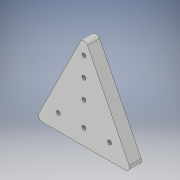
# Autodesk Inventor part: backsupportplate
Saved by Autodesk Inventor 2018 (Build 220112000, 112)
## iProperties
Created: 2018-07-30
Part Number: backsupportplate
Material: Generic
Document SubType Name: Modeling
Designer: Cole Tucker
Density: 1 g/cm^3
Appearance: Default
Author: Cole Tucker
Autodesk Inventor part; units mm, degrees
ref_plane "YZ Plane" through (0, 0, 0) normal (1, 0, 0) x (0, 1, 0)
ref_plane "XZ Plane" through (0, 0, 0) normal (0, 1, 0) x (-1, 0, 0)
ref_plane "XY Plane" through (0, 0, 0) normal (0, 0, 1) x (1, 0, 0)
sketch "Sketch1" plane through (0, 0, 0) normal (0, 0, 1) x (1, 0, 0)
  line L0 (0, 0) -> (0, 76.2)
  line L1 (0, 0) -> (32.9627, 0)
  line L2 (0, 0) -> (-32.9627, 0)
  line L3 (-35.8025, 4.5949) -> (-2.8398, 70.5204)
  line L4 (2.8398, 70.5204) -> (35.8025, 4.5949)
  arc A0 (-35.8025, 4.5949) -> (-32.9627, 0) centre (-32.9627, 3.175) ccw
  arc A1 (32.9627, 0) -> (35.8025, 4.5949) centre (32.9627, 3.175) ccw
  arc A2 (2.8398, 70.5204) -> (-2.8398, 70.5204) centre (0, 69.1005) ccw
  point P0 (38.1, 0)
  point P1 (-38.1, 0)
  dimension "d0" = 76.2
  dimension "d1" = 38.1
  dimension "d2" = 38.1
  dimension "d3" = 3.175
  constraints: 10 end point, 6 point on circle, 6 point on line, 6 tangent, 3 centre point, 2 equal radius, 2 horizontal, 1 vertical
  measures "d0" distance of L0.start L0.end
  measures "d1" distance of L0.start point (38.1, 0)
  measures "d2" distance of L0.start point (-38.1, 0)
  measures "d3" radius of A0
extrude "Extrusion1" add sketch "Sketch1" along normal blind 9.525
sketch "Sketch2" plane through (0, 0, 9.525) normal (0, 0, 1) x (1, 0, 0)
  arc A0 (2.8398, 70.5204) -> (-2.8398, 70.5204) centre (0, 69.1005) ccw projected
  line L0 (0, 72.2755) -> (0, 0)
  line L1 (0, 0) -> (0, 12.7)
  line L2 (0, 12.7) -> (-31.75, 12.7)
  line L3 (-2.8398, 70.5204) -> (-35.8025, 4.5949) projected
  line L4 (0, 12.7) -> (31.75, 12.7)
  line L5 (35.8025, 4.5949) -> (2.8398, 70.5204) projected
  line L6 (0, 12.7) -> (-20.32, 12.7) construction
  line L7 (0, 12.7) -> (20.32, 12.7) construction
  line L8 (0, 12.7) -> (0, 31.75)
  line L9 (0, 31.75) -> (0, 46.99)
  line L10 (0, 46.99) -> (0, 62.23)
  dimension "d6" = 12.7
  dimension "d7" = 20.32
  dimension "d8" = 20.32
  dimension "d9" = 19.05
  dimension "d10" = 15.24
  dimension "d11" = 15.24
  constraints: 18 end point, 8 point on line, 6 coincident, 1 horizontal, 1 perpendicular, 1 point on circle, 1 vertical
  measures "d6" distance of L0.end L1.end
  measures "d7" distance of L1.end L6.end
  measures "d8" distance of L1.end L7.end
  measures "d9" distance of L8.start L8.end
  measures "d10" distance of L8.end L9.end
  measures "d11" distance of L9.end L10.end
hole "Hole1" at (-20.32, 12.7, 9.525) at (0, 12.7, 9.525) at (20.32, 12.7, 9.525) at (0, 62.23, 9.525) at (0, 46.99, 9.525) at (0, 31.75, 9.525) direction (0, 0, -1) diameter 3.175 depth 25.4 tip angle 118
body "Solid1"
